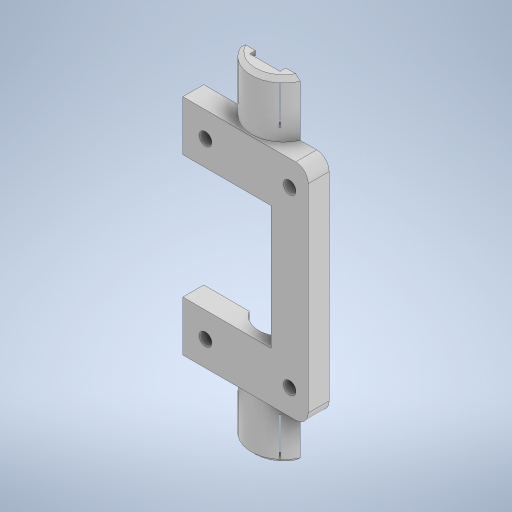
# Autodesk Inventor part: joný=gej
Saved by Autodesk Inventor 2024 (Build 280153000, 153)
## iProperties
Created: 2023-05-01
Part Number: joný=gej
Material: Všeobecné
Document SubType Name: Modeling
Designer: Simak
Density: 1 g/cm^3
Appearance: Výchozí
Author: Simak
Autodesk Inventor part; units mm, degrees
ref_plane "YZ Plane" through (0, 0, 0) normal (1, 0, 0) x (0, 1, 0)
ref_plane "XZ Plane" through (0, 0, 0) normal (0, 1, 0) x (-1, 0, 0)
ref_plane "XY Plane" through (0, 0, 0) normal (0, 0, 1) x (1, 0, 0)
sketch "Náčrt1" plane through (0, 0, 0) normal (0, 0, 1) x (1, 0, 0)
  line L0 (0, 0) -> (0, 26.75)
  line L1 (0, 26.75) -> (-30, 26.75)
  line L2 (-30, 26.75) -> (-30, 14.75)
  line L3 (-30, 14.75) -> (-8.875, 14.75)
  line L4 (-8.875, 14.75) -> (-8.875, 0)
  line L5 (-8.875, 0) -> (0, 0)
  circle A0 centre (-24.5625, 20.75) radius 1.5
  circle A1 centre (-4.4375, 20.75) radius 1.5
  line L6 (-19.125, 26.75) -> (-19.125, 14.75) construction
  dimension "d0" = 30
  dimension "d1" = 26.75
  dimension "d3" = 12
  dimension "d4" = 8.875
  dimension "d5" = 3
  dimension "d6" = 3
  dimension "d7" = 6
  dimension "d9" = 10.875
  dimension "d10" = 5.4375
  dimension "d11" = 4.4375
  constraints: 14 end point, 6 perpendicular, 2 centre point, 2 point on line, 1 horizontal alignment, 1 vertical
  measures "d0" distance of L0.end L1.end
  measures "d1" distance of L0.start L0.end
  measures "d3" distance of L1.end L2.end
  measures "d4" distance between parallel lines of L0 L4
  measures "d5" diameter of A0
  measures "d6" diameter of A1
  measures "d7" distance from line of L1 A0.centre
  measures "d9" distance between parallel lines of L2 L6
  measures "d10" distance from line of L2 A0.centre
  measures "d11" distance from line of L0 A1.centre
extrude "Vysunutí1" add sketch "Náčrt1" along normal blind 5
sketch "Náčrt2" plane through (-30, 26.75, 0) normal (0, 1, 0) x (1, 0, 0)
  circle A0 centre (16, 3.12) radius 6
  line L0 (30, 0) -> (0, 0) projected
  line L1 (21.125, 0) -> (21.125, -5) projected
  line L2 (30, -5) -> (0, -5) projected
  line L3 (10.875, -5) -> (10.875, 0)
  circle A1 centre (16, 3.12) radius 7.75
  point P0 (23.0942, 0)
  point P1 (8.9058, 0)
  dimension "d0" = 30
  dimension "d14" = 12
  dimension "d15" = 10.25
  dimension "d20" = 15.5
  constraints: 2 centre point, 2 end point, 2 point on circle, 2 point on line, 1 coincident, 1 parallel, 1 vertical
  measures "d14" diameter of A0
  measures "d15" distance between parallel lines of L3 L1
  measures "d20" diameter of A1
extrude "Vysunutí2" add sketch "Náčrt2" along normal blind 3 contours L3 A1 L0 | A0 L1 A1 L3 | L0 A1 L1
extrude "Vysunutí3" cut sketch "Náčrt2" against normal through all contours L0 A0 picked at (15.3305, -1.5618)
sketch "Náčrt4" plane through (-30, 29.75, 0) normal (0, 1, 0) x (1, 0, 0)
  line L0 (21.125, 0) -> (21.125, -2.88)
  line L1 (21.125, 0) -> (21.125, -5) projected
  arc A0 (10.875, 0) -> (21.125, 0) centre (16, 3.12) ccw projected
  line L2 (10.875, -2.88) -> (10.875, 0)
  line L3 (21.125, -2.88) -> (10.875, -2.88)
  arc A1 (8.9058, 0) -> (23.0942, 0) centre (16, 3.12) ccw projected
  line L4 (23.0942, 0) -> (21.125, 0) projected
  line L5 (10.875, 0) -> (8.9058, 0) projected
  point P0 (30, 0)
  point P1 (10.875, -2.6935)
  point P2 (21.125, -2.6935)
  point P3 (20.9054, -2.88)
  point P4 (11.0946, -2.88)
  point P5 (16, -2.88)
  constraints: 6 end point, 1 horizontal, 1 point on line, 1 tangent, 1 vertical
extrude "Vysunutí4" add sketch "Náčrt4" along normal blind 9.25 contours L4 A1 L0 | L3 A1 | L2 A1 L5
chamfer "Zkosení1" distance 0.25 angle 45 2 edges at (-16.9394, 29.75, 2.1107) (-11.0606, 29.75, 2.1107)
sketch "Náčrt6" plane through (-30, 39, 0) normal (0, 1, 0) x (1, 0, 0)
  arc A0 (21.125, -2.6935) -> (23.0942, 0) centre (16, 3.12) ccw projected
  arc A1 (20.9054, -2.88) -> (21.125, -2.6935) centre (16, 3.12) ccw projected
  arc A2 (11.0946, -2.88) -> (20.9054, -2.88) centre (16, 3.12) ccw projected
  arc A3 (8.9058, 0) -> (10.875, -2.6935) centre (16, 3.12) ccw projected
  arc A4 (10.875, -2.6935) -> (11.0946, -2.88) centre (16, 3.12) ccw projected
  line L0 (23.0942, 0) -> (21.125, 0) projected
  line L1 (10.875, 0) -> (8.9058, 0) projected
  line L2 (17.75, -2.88) -> (20.9054, -2.88) projected
  line L3 (11.0946, -2.88) -> (14.25, -2.88) projected
  line L4 (10.875, -0.4573) -> (10.875, -2.6935) projected
  line L5 (21.125, -2.6935) -> (21.125, -0.4573) projected
  line L6 (21.125, 0) -> (19.625, 0)
  line L7 (19.625, 0) -> (19.625, -1.38)
  line L8 (19.625, -1.38) -> (12.375, -1.38)
  line L9 (12.375, -1.38) -> (12.375, 0)
  line L10 (12.375, 0) -> (10.875, 0)
  point P0 (30, 0)
  dimension "d34" = 1.5
  dimension "d35" = 1.5
  dimension "d36" = 1.5
  constraints: 10 end point, 4 perpendicular, 1 horizontal, 1 point on line
  measures "d34" distance between parallel lines of L5 L7
  measures "d35" distance between parallel lines of L2 L8
  measures "d36" distance between parallel lines of L4 L9
extrude "Vysunutí5" add sketch "Náčrt6" along normal blind 1
chamfer "Zkosení2" distance 1 angle 45 1 edges at (-14, 40, 4.63)
mirror "Zrcadlit1" about plane through (-8.875, 0, 0) normal (0, -1, 0)
fillet "Zaoblení1" radius 3 2 edges at (0, 26.75, 2.5) (0, -26.75, 2.5)
